Autodesk Fusion 360 part; units mm, degrees
note: some values were not read from the file. Set by a fixed rule: which face or edge a step refers to.
(part 4 of 12)
  spline S14 degree 5 poles (-2.4466, 3.8949) (-2.4467, 3.8949) (-2.4468, 3.8951) (-2.447, 3.8954) (-2.4473, 3.8958) (-2.4477, 3.8965) (-2.4482, 3.8972) (-2.4488, 3.8981) (-2.4495, 3.899) (-2.4502, 3.9) (-2.451, 3.9011) (-2.4518, 3.9023) (-2.4528, 3.9036) (-2.4538, 3.905) (-2.4549, 3.9065) (-2.456, 3.908) (-2.4572, 3.9096) (-2.4585, 3.9113) (-2.4599, 3.9131) (-2.4613, 3.9149) (-2.4629, 3.9168) (-2.4644, 3.9188) (-2.4661, 3.9208) (-2.4678, 3.9229) (-2.4696, 3.9251) (-2.4715, 3.9274) (-2.4734, 3.9297) (-2.4754, 3.9321) (-2.4775, 3.9345) (-2.4797, 3.937) (-2.4819, 3.9395) (-2.4842, 3.9421) (-2.4865, 3.9448) (-2.489, 3.9475) (-2.4915, 3.9503) (-2.4941, 3.9531) (-2.4967, 3.956) (-2.4994, 3.9589) (-2.5022, 3.9619) (-2.5051, 3.9649) (-2.508, 3.968) (-2.511, 3.9711) (-2.5141, 3.9742) (-2.5172, 3.9774) (-2.5205, 3.9807) (-2.5237, 3.9839) (-2.5271, 3.9873) (-2.5305, 3.9906) (-2.534, 3.994) (-2.5376, 3.9975) (-2.5412, 4.0009) (-2.5449, 4.0044) (-2.5487, 4.008) (-2.5525, 4.0116) (-2.5565, 4.0152) (-2.5604, 4.0188) (-2.5645, 4.0225) (-2.5686, 4.0262) (-2.5728, 4.0299) (-2.577, 4.0337) (-2.5814, 4.0375) (-2.5858, 4.0413) (-2.5902, 4.0451) (-2.5948, 4.049) (-2.5994, 4.0529) (-2.604, 4.0568) (-2.6088, 4.0607) (-2.6136, 4.0647) (-2.6184, 4.0686) (-2.6234, 4.0726) (-2.6284, 4.0767) (-2.6335, 4.0807) (-2.6386, 4.0848) (-2.6438, 4.0888) (-2.6491, 4.0929) (-2.6544, 4.097) (-2.6598, 4.1012) (-2.6653, 4.1053) (-2.6708, 4.1095) (-2.6764, 4.1136) (-2.6821, 4.1178) (-2.6878, 4.122) (-2.6936, 4.1262) (-2.6995, 4.1304) (-2.7055, 4.1346) (-2.7115, 4.1389) (-2.7175, 4.1431) (-2.7236, 4.1474) (-2.7298, 4.1516) (-2.7361, 4.1559) (-2.7424, 4.1602) (-2.7488, 4.1645) (-2.7553, 4.1688) (-2.7618, 4.1731) (-2.7684, 4.1774) (-2.775, 4.1817) (-2.7817, 4.186) (-2.7885, 4.1903) (-2.7953, 4.1946) (-2.8022, 4.1989) (-2.8092, 4.2032) (-2.8162, 4.2075) (-2.8233, 4.2119) (-2.8304, 4.2162) (-2.8376, 4.2205) (-2.8449, 4.2248) (-2.8522, 4.2291) (-2.8596, 4.2334) (-2.8671, 4.2377) (-2.8746, 4.2421) (-2.8822, 4.2464) (-2.8898, 4.2507) (-2.8975, 4.2549) (-2.9053, 4.2592) (-2.9131, 4.2635) (-2.921, 4.2678) (-2.9289, 4.2721) (-2.9369, 4.2763) (-2.945, 4.2806) (-2.9531, 4.2848) (-2.9613, 4.2891) (-2.9695, 4.2933) (-2.9778, 4.2975) (-2.9862, 4.3018) (-2.9946, 4.306) (-3.003, 4.3102) (-3.0116, 4.3143) (-3.0202, 4.3185) (-3.0288, 4.3227) (-3.0375, 4.3268) (-3.0463, 4.331) (-3.0551, 4.3351) (-3.064, 4.3392) (-3.0729, 4.3433) (-3.0819, 4.3474) (-3.0909, 4.3514) (-3.1, 4.3555) (-3.1092, 4.3595) (-3.1184, 4.3635) (-3.1277, 4.3676) (-3.137, 4.3715) (-3.1464, 4.3755) (-3.1558, 4.3795) (-3.1653, 4.3834) (-3.1749, 4.3873) (-3.1845, 4.3912) (-3.1941, 4.3951) (-3.2038, 4.399) (-3.2136, 4.4028) (-3.2234, 4.4067) (-3.2333, 4.4105) (-3.2432, 4.4143) (-3.2532, 4.418) (-3.2632, 4.4218) (-3.2733, 4.4255) (-3.2834, 4.4292) (-3.2936, 4.4329) (-3.3039, 4.4365) (-3.3141, 4.4402) (-3.3245, 4.4438) (-3.3349, 4.4474) (-3.3453, 4.4509) (-3.3558, 4.4545) (-3.3664, 4.458) (-3.377, 4.4615) (-3.3876, 4.465) (-3.3983, 4.4684) (-3.4091, 4.4718) (-3.4199, 4.4752) (-3.4307, 4.4786) (-3.4416, 4.4819) (-3.4526, 4.4853) (-3.4636, 4.4886) (-3.4746, 4.4918) (-3.4857, 4.495) (-3.4969, 4.4983) (-3.508, 4.5014) (-3.5193, 4.5046) (-3.5306, 4.5077) (-3.5419, 4.5108) (-3.5533, 4.5139) (-3.5647, 4.5169) (-3.5762, 4.5199) (-3.5877, 4.5229) (-3.5993, 4.5258) (-3.6109, 4.5287) (-3.6226, 4.5316) (-3.6343, 4.5345) (-3.646, 4.5373) (-3.6578, 4.5401) (-3.6697, 4.5429) (-3.6816, 4.5456) (-3.6935, 4.5483) (-3.7055, 4.5509) (-3.7175, 4.5536) (-3.7296, 4.5562) (-3.7417, 4.5587) (-3.7538, 4.5613) (-3.766, 4.5638) (-3.7783, 4.5662) (-3.7906, 4.5687) (-3.8029, 4.5711) (-3.8153, 4.5734) (-3.8277, 4.5757) (-3.8401, 4.578) (-3.8526, 4.5803) (-3.8652, 4.5825) (-3.8778, 4.5847) (-3.8904, 4.5868) (-3.903, 4.589) (-3.9157, 4.591) (-3.9285, 4.5931) (-3.9413, 4.5951) (-3.9541, 4.597) (-3.967, 4.599) (-3.9799, 4.6009) (-3.9928, 4.6027) (-4.0058, 4.6045) (-4.0188, 4.6063) (-4.0319, 4.6081) (-4.045, 4.6098) (-4.0582, 4.6114) (-4.0713, 4.6131) (-4.0846, 4.6146) (-4.0978, 4.6162) (-4.1111, 4.6177) (-4.1244, 4.6192) (-4.1378, 4.6206) (-4.1512, 4.622) (-4.1647, 4.6233) (-4.1782, 4.6246) (-4.1917, 4.6259) (-4.2052, 4.6271) (-4.2188, 4.6283) (-4.2324, 4.6295) (-4.2461, 4.6306) (-4.2598, 4.6316) (-4.2735, 4.6327) (-4.2873, 4.6336) (-4.3011, 4.6346) (-4.3149, 4.6355) (-4.326, 4.6362) (-4.3344, 4.6367) (-4.3399, 4.637) (-4.3427, 4.6371) knots 0 0 0 0 0 0 0.00416667 0.00833333 0.0125 0.01666667 0.02083333 0.025 0.02916667 0.03333333 0.0375 0.04166667 0.04583333 0.05 0.05416667 0.05833333 0.0625 0.06666667 0.07083333 0.075 0.07916667 0.08333333 0.0875 0.09166667 0.09583333 0.1 0.10416667 0.10833333 0.1125 0.11666667 0.12083333 0.125 0.12916667 0.13333333 0.1375 0.14166667 0.14583333 0.15 0.15416667 0.15833333 0.1625 0.16666667 0.17083333 0.175 0.17916667 0.18333333 0.1875 0.19166667 0.19583333 0.2 0.20416667 0.20833333 0.2125 0.21666667 0.22083333 0.225 0.22916667 0.23333333 0.2375 0.24166667 0.24583333 0.25 0.25416667 0.25833333 0.2625 0.26666667 0.27083333 0.275 0.27916667 0.28333333 0.2875 0.29166667 0.29583333 0.3 0.30416667 0.30833333 0.3125 0.31666667 0.32083333 0.325 0.32916667 0.33333333 0.3375 0.34166667 0.34583333 0.35 0.35416667 0.35833333 0.3625 0.36666667 0.37083333 0.375 0.37916667 0.38333333 0.3875 0.39166667 0.39583333 0.4 0.40416667 0.40833333 0.4125 0.41666667 0.42083333 0.425 0.42916667 0.43333333 0.4375 0.44166667 0.44583333 0.45 0.45416667 0.45833333 0.4625 0.46666667 0.47083333 0.475 0.47916667 0.48333333 0.4875 0.49166667 0.49583333 0.5 0.50416667 0.50833333 0.5125 0.51666667 0.52083333 0.525 0.52916667 0.53333333 0.5375 0.54166667 0.54583333 0.55 0.55416667 0.55833333 0.5625 0.56666667 0.57083333 0.575 0.57916667 0.58333333 0.5875 0.59166667 0.59583333 0.6 0.60416667 0.60833333 0.6125 0.61666667 0.62083333 0.625 0.62916667 0.63333333 0.6375 0.64166667 0.64583333 0.65 0.65416667 0.65833333 0.6625 0.66666667 0.67083333 0.675 0.67916667 0.68333333 0.6875 0.69166667 0.69583333 0.7 0.70416667 0.70833333 0.7125 0.71666667 0.72083333 0.725 0.72916667 0.73333333 0.7375 0.74166667 0.74583333 0.75 0.75416667 0.75833333 0.7625 0.76666667 0.77083333 0.775 0.77916667 0.78333333 0.7875 0.79166667 0.79583333 0.8 0.80416667 0.80833333 0.8125 0.81666667 0.82083333 0.825 0.82916667 0.83333333 0.8375 0.84166667 0.84583333 0.85 0.85416667 0.85833333 0.8625 0.86666667 0.87083333 0.875 0.87916667 0.88333333 0.8875 0.89166667 0.89583333 0.9 0.90416667 0.90833333 0.9125 0.91666667 0.92083333 0.925 0.92916667 0.93333333 0.9375 0.94166667 0.94583333 0.95 0.95416667 0.95833333 0.9625 0.96666667 0.97083333 0.975 0.97916667 0.98333333 0.9875 0.99166667 0.99583333 1 1 1 1 1 1
  arc A15 (-4.3427, 4.6371) -> (-4.6371, 4.3427) centre (0, 0) ccw
  spline S15 degree 5 poles (-4.6371, 4.3427) (-4.637, 4.3399) (-4.6367, 4.3344) (-4.6362, 4.326) (-4.6355, 4.3149) (-4.6346, 4.3011) (-4.6336, 4.2873) (-4.6327, 4.2735) (-4.6316, 4.2598) (-4.6306, 4.2461) (-4.6295, 4.2324) (-4.6283, 4.2188) (-4.6271, 4.2052) (-4.6259, 4.1917) (-4.6246, 4.1782) (-4.6233, 4.1647) (-4.622, 4.1512) (-4.6206, 4.1378) (-4.6192, 4.1244) (-4.6177, 4.1111) (-4.6162, 4.0978) (-4.6146, 4.0846) (-4.6131, 4.0713) (-4.6114, 4.0582) (-4.6098, 4.045) (-4.6081, 4.0319) (-4.6063, 4.0188) (-4.6045, 4.0058) (-4.6027, 3.9928) (-4.6009, 3.9799) (-4.599, 3.967) (-4.597, 3.9541) (-4.5951, 3.9413) (-4.5931, 3.9285) (-4.591, 3.9157) (-4.589, 3.903) (-4.5868, 3.8904) (-4.5847, 3.8778) (-4.5825, 3.8652) (-4.5803, 3.8526) (-4.578, 3.8401) (-4.5757, 3.8277) (-4.5734, 3.8153) (-4.5711, 3.8029) (-4.5687, 3.7906) (-4.5662, 3.7783) (-4.5638, 3.766) (-4.5613, 3.7538) (-4.5587, 3.7417) (-4.5562, 3.7296) (-4.5536, 3.7175) (-4.5509, 3.7055) (-4.5483, 3.6935) (-4.5456, 3.6816) (-4.5429, 3.6697) (-4.5401, 3.6578) (-4.5373, 3.646) (-4.5345, 3.6343) (-4.5316, 3.6226) (-4.5287, 3.6109) (-4.5258, 3.5993) (-4.5229, 3.5877) (-4.5199, 3.5762) (-4.5169, 3.5647) (-4.5139, 3.5533) (-4.5108, 3.5419) (-4.5077, 3.5306) (-4.5046, 3.5193) (-4.5014, 3.508) (-4.4983, 3.4969) (-4.495, 3.4857) (-4.4918, 3.4746) (-4.4886, 3.4636) (-4.4853, 3.4526) (-4.4819, 3.4416) (-4.4786, 3.4307) (-4.4752, 3.4199) (-4.4718, 3.4091) (-4.4684, 3.3983) (-4.465, 3.3876) (-4.4615, 3.377) (-4.458, 3.3664) (-4.4545, 3.3558) (-4.4509, 3.3453) (-4.4474, 3.3349) (-4.4438, 3.3245) (-4.4402, 3.3141) (-4.4365, 3.3039) (-4.4329, 3.2936) (-4.4292, 3.2834) (-4.4255, 3.2733) (-4.4218, 3.2632) (-4.418, 3.2532) (-4.4143, 3.2432) (-4.4105, 3.2333) (-4.4067, 3.2234) (-4.4028, 3.2136) (-4.399, 3.2038) (-4.3951, 3.1941) (-4.3912, 3.1845) (-4.3873, 3.1749) (-4.3834, 3.1653) (-4.3795, 3.1558) (-4.3755, 3.1464) (-4.3715, 3.137) (-4.3676, 3.1277) (-4.3635, 3.1184) (-4.3595, 3.1092) (-4.3555, 3.1) (-4.3514, 3.0909) (-4.3474, 3.0819) (-4.3433, 3.0729) (-4.3392, 3.064) (-4.3351, 3.0551) (-4.331, 3.0463) (-4.3268, 3.0375) (-4.3227, 3.0288) (-4.3185, 3.0202) (-4.3143, 3.0116) (-4.3102, 3.003) (-4.306, 2.9946) (-4.3018, 2.9862) (-4.2975, 2.9778) (-4.2933, 2.9695) (-4.2891, 2.9613) (-4.2848, 2.9531) (-4.2806, 2.945) (-4.2763, 2.9369) (-4.2721, 2.9289) (-4.2678, 2.921) (-4.2635, 2.9131) (-4.2592, 2.9053) (-4.2549, 2.8975) (-4.2507, 2.8898) (-4.2464, 2.8822) (-4.2421, 2.8746) (-4.2377, 2.8671) (-4.2334, 2.8596) (-4.2291, 2.8522) (-4.2248, 2.8449) (-4.2205, 2.8376) (-4.2162, 2.8304) (-4.2119, 2.8233) (-4.2075, 2.8162) (-4.2032, 2.8092) (-4.1989, 2.8022) (-4.1946, 2.7953) (-4.1903, 2.7885) (-4.186, 2.7817) (-4.1817, 2.775) (-4.1774, 2.7684) (-4.1731, 2.7618) (-4.1688, 2.7553) (-4.1645, 2.7488) (-4.1602, 2.7424) (-4.1559, 2.7361) (-4.1516, 2.7298) (-4.1474, 2.7236) (-4.1431, 2.7175) (-4.1389, 2.7115) (-4.1346, 2.7055) (-4.1304, 2.6995) (-4.1262, 2.6936) (-4.122, 2.6878) (-4.1178, 2.6821) (-4.1136, 2.6764) (-4.1095, 2.6708) (-4.1053, 2.6653) (-4.1012, 2.6598) (-4.097, 2.6544) (-4.0929, 2.6491) (-4.0888, 2.6438) (-4.0848, 2.6386) (-4.0807, 2.6335) (-4.0767, 2.6284) (-4.0726, 2.6234) (-4.0686, 2.6184) (-4.0647, 2.6136) (-4.0607, 2.6088) (-4.0568, 2.604) (-4.0529, 2.5994) (-4.049, 2.5948) (-4.0451, 2.5902) (-4.0413, 2.5858) (-4.0375, 2.5814) (-4.0337, 2.577) (-4.0299, 2.5728) (-4.0262, 2.5686) (-4.0225, 2.5645) (-4.0188, 2.5604) (-4.0152, 2.5565) (-4.0116, 2.5525) (-4.008, 2.5487) (-4.0044, 2.5449) (-4.0009, 2.5412) (-3.9975, 2.5376) (-3.994, 2.534) (-3.9906, 2.5305) (-3.9873, 2.5271) (-3.9839, 2.5237) (-3.9807, 2.5205) (-3.9774, 2.5172) (-3.9742, 2.5141) (-3.9711, 2.511) (-3.968, 2.508) (-3.9649, 2.5051) (-3.9619, 2.5022) (-3.9589, 2.4994) (-3.956, 2.4967) (-3.9531, 2.4941) (-3.9503, 2.4915) (-3.9475, 2.489) (-3.9448, 2.4865) (-3.9421, 2.4842) (-3.9395, 2.4819) (-3.937, 2.4797) (-3.9345, 2.4775) (-3.9321, 2.4754) (-3.9297, 2.4734) (-3.9274, 2.4715) (-3.9251, 2.4696) (-3.9229, 2.4678) (-3.9208, 2.4661) (-3.9188, 2.4644) (-3.9168, 2.4629) (-3.9149, 2.4613) (-3.9131, 2.4599) (-3.9113, 2.4585) (-3.9096, 2.4572) (-3.908, 2.456) (-3.9065, 2.4549) (-3.905, 2.4538) (-3.9036, 2.4528) (-3.9023, 2.4518) (-3.9011, 2.451) (-3.9, 2.4502) (-3.899, 2.4495) (-3.8981, 2.4488) (-3.8972, 2.4482) (-3.8965, 2.4477) (-3.8958, 2.4473) (-3.8954, 2.447) (-3.8951, 2.4468) (-3.8949, 2.4467) (-3.8949, 2.4466) knots -1 -1 -1 -1 -1 -1 -0.99583333 -0.99166667 -0.9875 -0.98333333 -0.97916667 -0.975 -0.97083333 -0.96666667 -0.9625 -0.95833333 -0.95416667 -0.95 -0.94583333 -0.94166667 -0.9375 -0.93333333 -0.92916667 -0.925 -0.92083333 -0.91666667 -0.9125 -0.90833333 -0.90416667 -0.9 -0.89583333 -0.89166667 -0.8875 -0.88333333 -0.87916667 -0.875 -0.87083333 -0.86666667 -0.8625 -0.85833333 -0.85416667 -0.85 -0.84583333 -0.84166667 -0.8375 -0.83333333 -0.82916667 -0.825 -0.82083333 -0.81666667 -0.8125 -0.80833333 -0.80416667 -0.8 -0.79583333 -0.79166667 -0.7875 -0.78333333 -0.77916667 -0.775 -0.77083333 -0.76666667 -0.7625 -0.75833333 -0.75416667 -0.75 -0.74583333 -0.74166667 -0.7375 -0.73333333 -0.72916667 -0.725 -0.72083333 -0.71666667 -0.7125 -0.70833333 -0.70416667 -0.7 -0.69583333 -0.69166667 -0.6875 -0.68333333 -0.67916667 -0.675 -0.67083333 -0.66666667 -0.6625 -0.65833333 -0.65416667 -0.65 -0.64583333 -0.64166667 -0.6375 -0.63333333 -0.62916667 -0.625 -0.62083333 -0.61666667 -0.6125 -0.60833333 -0.60416667 -0.6 -0.59583333 -0.59166667 -0.5875 -0.58333333 -0.57916667 -0.575 -0.57083333 -0.56666667 -0.5625 -0.55833333 -0.55416667 -0.55 -0.54583333 -0.54166667 -0.5375 -0.53333333 -0.52916667 -0.525 -0.52083333 -0.51666667 -0.5125 -0.50833333 -0.50416667 -0.5 -0.49583333 -0.49166667 -0.4875 -0.48333333 -0.47916667 -0.475 -0.47083333 -0.46666667 -0.4625 -0.45833333 -0.45416667 -0.45 -0.44583333 -0.44166667 -0.4375 -0.43333333 -0.42916667 -0.425 -0.42083333 -0.41666667 -0.4125 -0.40833333 -0.40416667 -0.4 -0.39583333 -0.39166667 -0.3875 -0.38333333 -0.37916667 -0.375 -0.37083333 -0.36666667 -0.3625 -0.35833333 -0.35416667 -0.35 -0.34583333 -0.34166667 -0.3375 -0.33333333 -0.32916667 -0.325 -0.32083333 -0.31666667 -0.3125 -0.30833333 -0.30416667 -0.3 -0.29583333 -0.29166667 -0.2875 -0.28333333 -0.27916667 -0.275 -0.27083333 -0.26666667 -0.2625 -0.25833333 -0.25416667 -0.25 -0.24583333 -0.24166667 -0.2375 -0.23333333 -0.22916667 -0.225 -0.22083333 -0.21666667 -0.2125 -0.20833333 -0.20416667 -0.2 -0.19583333 -0.19166667 -0.1875 -0.18333333 -0.17916667 -0.175 -0.17083333 -0.16666667 -0.1625 -0.15833333 -0.15416667 -0.15 -0.14583333 -0.14166667 -0.1375 -0.13333333 -0.12916667 -0.125 -0.12083333 -0.11666667 -0.1125 -0.10833333 -0.10416667 -0.1 -0.09583333 -0.09166667 -0.0875 -0.08333333 -0.07916667 -0.075 -0.07083333 -0.06666667 -0.0625 -0.05833333 -0.05416667 -0.05 -0.04583333 -0.04166667 -0.0375 -0.03333333 -0.02916667 -0.025 -0.02083333 -0.01666667 -0.0125 -0.00833333 -0.00416667 0 0 0 0 0 0
  line L30 (-3.8949, 2.4466) -> (-3.8941, 2.4462)
  line L31 (-3.8941, 2.4462) -> (-3.1172, 1.9582)
  circle A16 centre (0, 0) radius 2.925
  line L32 (3, 1) -> (-3, 1)
  line L33 (-3, 1) -> (-3, -1)
  line L34 (-3, -1) -> (3, -1)
  line L35 (3, -1) -> (3, 1)
  line L36 (3, 1) -> (-3, -1) construction
  line L37 (-3, 1) -> (3, -1) construction
  line L38 (2.9, 0.9) -> (-2.9, 0.9)
  line L39 (-2.9, 0.9) -> (-2.9, -0.9)
  line L40 (-2.9, -0.9) -> (2.9, -0.9)
  line L41 (2.9, -0.9) -> (2.9, 0.9)
  line L42 (0, -1) -> (0, 1)
  dimension "d32" = 5.85
  dimension "d37" = 6
  dimension "d38" = 2
  dimension "d39" = -0.1
  constraint concentric A0 A16
  constraint horizontal L32
  constraint perpendicular L32 L33
  constraint parallel L32 L34
  constraint parallel L33 L35
  constraint coincident L36 A0.centre
  constraint coincident L37 A0.centre
  constraint coincident A0.centre A1.centre
  constraint midpoint L34 L42.start
  constraint midpoint L32 L42.end
  measures "d32" diameter of A16
  measures "d37" distance of L33.end L34.end
  measures "d38" distance of L32.end L33.end
extrude "Extrude4" cut sketch "Sketch2 (3)" against normal blind 5 contours A16 L32 L38 L42 | A16 L34 L40 L42 | A16 L32 | A16 L38 L39 L40 L42 | A16 L32 L38 L42 | A16 L34 | A16 L34 L40 L42 | A16 L39 bodies 1 in component "Component"
extrude "Extrude3" cut sketch "Sketch2 (3)" against normal blind 5 contours A16 L32 L38 L42 | A16 L34 L40 L42 | A16 L32 | A16 L38 L39 L40 L42 | A16 L32 L38 L42 | A16 L34 | A16 L34 L40 L42 | A16 L39 bodies 10 in component "Component'"
component "Component" placed x (1, 0, 0) y (0, 1, 0) z (0, 0, 1) at (30, 0, 0)
component "Component'" placed x (1, 0, 0) y (0, 1, 0) z (0, 0, 1) at (0, 0, 0)
component "Component" placed x (1, 0, 0) y (0, 1, 0) z (0, 0, 1) at (45, 0, 0)
component "Component'" placed x (1, 0, 0) y (0, 1, 0) z (0, 0, 1) at (-46, 0, 0)

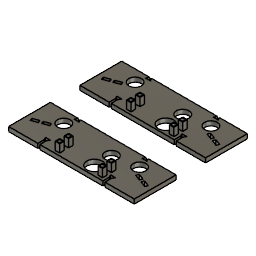
design "card-shuffler-side-plates"
part number: 2026-07-14-13-37-18-342
part number: 2026-07-29-15-30-40-937
Autodesk Fusion 360 part; units mm, degrees
sketch "Sketch1" plane through (0, 0, 0) normal (0, 0, 1) x (1, 0, 0)
  line L0 (0, 0) -> (81, 0)
  line L1 (81, 0) -> (81, 103)
  line L2 (81, 103) -> (0, 103)
  line L3 (0, 103) -> (0, 0)
  line L4 (76, 98) -> (5, 98)
  line L5 (5, 98) -> (5, 5)
  line L6 (5, 5) -> (76, 5)
  line L7 (76, 5) -> (76, 98)
  line L8 (76, 98) -> (5, 5) construction
  line L9 (5, 98) -> (76, 5) construction
  line L10 (81, 0) -> (111, 0)
  line L11 (111, 0) -> (111, 5)
  line L12 (111, 5) -> (81, 5)
  line L13 (81, 5) -> (81, 0)
  line L14 (0, 0) -> (-30, 0)
  line L15 (-30, 0) -> (-30, 5)
  line L16 (-30, 5) -> (0, 5)
  line L17 (0, 5) -> (0, 0)
  line L18 (81, 103) -> (111, 103)
  line L19 (111, 103) -> (111, 98)
  line L20 (111, 98) -> (81, 98)
  line L21 (81, 98) -> (81, 103)
  line L22 (0, 103) -> (-30, 103)
  line L23 (-30, 103) -> (-30, 98)
  line L24 (-30, 98) -> (0, 98)
  line L25 (0, 98) -> (0, 103)
  line L26 (76, 51.5) -> (76, 45)
  line L27 (76, 45) -> (81, 45)
  line L28 (81, 45) -> (81, 58)
  line L29 (81, 58) -> (76, 58)
  line L30 (76, 58) -> (76, 45)
  line L31 (0, 58) -> (5, 58)
  line L32 (5, 58) -> (5, 45)
  line L33 (5, 45) -> (0, 45)
  line L34 (0, 45) -> (0, 58)
  line L35 (81, 98) -> (111, 98)
  line L36 (111, 98) -> (111, 5)
  line L37 (111, 5) -> (81, 5)
  line L38 (81, 5) -> (81, 98)
  line L39 (-30, 98) -> (0, 98)
  line L40 (0, 98) -> (0, 5)
  line L41 (0, 5) -> (-30, 5)
  line L42 (-30, 5) -> (-30, 98)
  line L43 (76, 58) -> (108, 58)
  line L44 (108, 58) -> (108, 45)
  line L45 (108, 45) -> (76, 45)
  line L46 (76, 45) -> (76, 58)
  line L47 (5, 45) -> (-27, 45)
  line L48 (-27, 45) -> (-27, 58)
  line L49 (-27, 58) -> (5, 58)
  line L50 (5, 58) -> (5, 45)
  line L51 (76, 98) -> (81, 98)
  line L52 (5, 98) -> (0, 98)
  line L53 (0, 5) -> (5, 5)
  line L54 (76, 5) -> (81, 5)
  point P0 (40.5, 51.5)
  dimension "d1" = 81
  dimension "d2" = 103
  dimension "d3" = 71
  dimension "d4" = 93
  dimension "d7" = 6.5
  dimension "d8" = 32
  dimension "d9" = 13
  dimension "d14" = 30
  dimension "d15" = 30
  dimension "d16" = 30
  dimension "d17" = 30
  constraint horizontal L0
  constraint vertical L1
  constraint horizontal L2
  constraint vertical L3
  constraint coincident L0.start L3.end
  constraint horizontal L4
  constraint perpendicular L4 L5
  constraint parallel L4 L6
  constraint parallel L5 L7
  constraint coincident L8 P0
  constraint coincident L9 P0
  constraint horizontal L10
  constraint vertical L11
  constraint horizontal L12
  constraint vertical L13
  constraint horizontal L14
  constraint vertical L15
  constraint horizontal L16
  constraint vertical L17
  constraint horizontal L18
  constraint vertical L19
  constraint horizontal L20
  constraint vertical L21
  constraint horizontal L22
  constraint vertical L23
  constraint horizontal L24
  constraint vertical L25
  constraint midpoint L7 L26.start
  constraint parallel L7 L26
  constraint horizontal L27
  constraint vertical L28
  constraint horizontal L29
  constraint vertical L30
  constraint coincident L1 L28.end
  constraint horizontal L31
  constraint vertical L32
  constraint horizontal L33
  constraint vertical L34
  constraint coincident L5 L32.end
  constraint coincident L3 L31.start
  constraint horizontal L35
  constraint vertical L36
  constraint horizontal L37
  constraint vertical L38
  constraint horizontal L39
  constraint vertical L40
  constraint horizontal L41
  constraint vertical L42
  constraint horizontal L43
  constraint vertical L44
  constraint horizontal L45
  constraint vertical L46
  constraint horizontal L47
  constraint vertical L48
  constraint horizontal L49
  constraint vertical L50
  measures "d1" distance of L0.start L0.end
  measures "d2" distance of L0.start L2.end
  measures "d3" distance of L5.end L6.end
  measures "d4" distance of L4.end L5.end
  measures "d7" distance of L26.start L26.end
  measures "d8" distance of L32.end L47.end
  measures "d9" distance of L32.end L31.end
  measures "d14" distance of L36 L38
  measures "d15" distance of L3 L42
  measures "d16" distance of L15 L17
  measures "d17" distance of L19 L21
extrude "Extrude1" add sketch "Sketch1" along normal blind 62 contours L0 L1 L3 L6 L13 L17 L53 L54 | L3 L14 L15 L16 L17 L41 | L1 L10 L11 L12 L13 L37 makes body 1
sketch "Sketch2" plane through (0, 0, 62) normal (0, 0, 1) x (-1, 0, 0)
  line L0 (-76, -98) -> (-81, -98)
  line L1 (-5, -98) -> (0, -98)
  line L2 (0, -5) -> (-5, -5)
  line L3 (40, -98) -> (-121, -98)
  line L4 (-121, -98) -> (-121, -103)
  line L5 (-121, -103) -> (40, -103)
  line L6 (40, -103) -> (40, -98)
  line L7 (40, -5) -> (-121, -5)
  line L8 (-121, -5) -> (-121, 0)
  line L9 (-121, 0) -> (40, 0)
  line L10 (40, 0) -> (40, -5)
  line L11 (0, -5) -> (30, -5)
  line L12 (30, -5) -> (30, 0)
  line L13 (30, 0) -> (-111, 0)
  line L14 (-111, 0) -> (-111, -5)
  line L15 (-111, -5) -> (-81, -5)
  line L16 (-81, -5) -> (-76, -5)
  line L17 (-76, -5) -> (-5, -5)
  line L18 (-5, -5) -> (0, -5)
  constraint horizontal L3
  constraint vertical L4
  constraint horizontal L5
  constraint vertical L6
  constraint horizontal L7
  constraint vertical L8
  constraint horizontal L9
  constraint vertical L10
sketch "Sketch5" plane through (0, 0, 0) normal (0, -1, 0) x (1, 0, 0)
  line L0 (-30, 0) -> (111, 0)
  line L1 (111, 0) -> (111, 62)
  line L2 (111, 62) -> (-30, 62)
  line L3 (-30, 62) -> (-30, 0)
  line L4 (40.5, 62) -> (40.5, 0)
  circle A0 centre (-2, 28) radius 7.05
  circle A1 centre (56, 51.6) radius 8.5
  circle A2 centre (70, 46.6) radius 1.95
  circle A3 centre (70, 56.6) radius 1.95
  line L5 (72.5, 59.1) -> (67.5, 59.1)
  line L6 (67.5, 59.1) -> (67.5, 54.1)
  line L7 (67.5, 54.1) -> (72.5, 54.1)
  line L8 (72.5, 54.1) -> (72.5, 59.1)
  line L9 (72.5, 59.1) -> (67.5, 54.1) construction
  line L10 (67.5, 59.1) -> (72.5, 54.1) construction
  line L11 (72.5, 49.1) -> (67.5, 49.1)
  line L12 (67.5, 49.1) -> (67.5, 44.1)
  line L13 (67.5, 44.1) -> (72.5, 44.1)
  line L14 (72.5, 44.1) -> (72.5, 49.1)
  line L15 (72.5, 49.1) -> (67.5, 44.1) construction
  line L16 (67.5, 49.1) -> (72.5, 44.1) construction
  circle A4 centre (83, 28) radius 7.05
  line L17 (0, 0) -> (80, 0)
  line L18 (80, 0) -> (80, 15)
  line L19 (80, 15) -> (0, 15)
  line L20 (0, 15) -> (0, 0)
  line L21 (0, 15) -> (-30, 15)
  line L22 (-30, 15) -> (-30, 0)
  line L23 (-30, 0) -> (0, 0)
  line L24 (0, 0) -> (0, 15)
  line L25 (80, 15) -> (111, 15)
  line L26 (111, 15) -> (111, 0)
  line L27 (111, 0) -> (80, 0)
  line L28 (80, 0) -> (80, 15)
  line L29 (0, 15) -> (5, 15)
  line L30 (5, 15) -> (5, 18)
  line L31 (5, 18) -> (0, 18)
  line L32 (0, 18) -> (0, 15)
  line L33 (80, 15) -> (75, 15)
  line L34 (81, 18) -> (76, 18)
  line L35 (76, 18) -> (76, 15)
  line L36 (76, 15) -> (81, 15)
  line L37 (81, 15) -> (81, 18)
  line L38 (-7.7431, 38.0574) -> (-14.3209, 40.4516)
  line L39 (-7.7431, 38.0574) -> (-8.7691, 35.2384)
  line L40 (-8.7691, 35.2384) -> (-15.347, 37.6325)
  line L41 (-15.347, 37.6325) -> (-14.3209, 40.4516)
  line L42 (-17.1354, 41.4902) -> (-23.7133, 43.8843)
  line L43 (-17.1354, 41.4902) -> (-18.1615, 38.6711)
  line L44 (-18.1615, 38.6711) -> (-24.7393, 41.0652)
  line L45 (-24.7393, 41.0652) -> (-23.7133, 43.8843)
  line L46 (105.7393, 41.0652) -> (104.7133, 43.8843)
  line L47 (99.1615, 38.6711) -> (105.7393, 41.0652)
  line L48 (96.347, 37.6325) -> (95.3209, 40.4516)
  line L49 (88.7431, 38.0574) -> (95.3209, 40.4516)
  line L50 (98.1354, 41.4902) -> (99.1615, 38.6711)
  line L51 (98.1354, 41.4902) -> (104.7133, 43.8843)
  line L52 (89.7691, 35.2384) -> (96.347, 37.6325)
  line L53 (88.7431, 38.0574) -> (89.7691, 35.2384)
  line L54 (19.5, 59.1) -> (19.5, 54.1)
  line L55 (24.5, 49.1) -> (19.5, 49.1)
  line L56 (24.5, 44.1) -> (24.5, 49.1)
  line L57 (19.5, 44.1) -> (24.5, 44.1)
  line L58 (19.5, 49.1) -> (24.5, 44.1) construction
  line L59 (24.5, 59.1) -> (19.5, 59.1)
  line L60 (24.5, 54.1) -> (24.5, 59.1)
  line L61 (19.5, 54.1) -> (24.5, 54.1)
  line L62 (24.5, 59.1) -> (19.5, 54.1) construction
  circle A5 centre (22, 56.6) radius 1.95
  line L63 (19.5, 49.1) -> (19.5, 44.1)
  line L64 (19.5, 59.1) -> (24.5, 54.1) construction
  circle A6 centre (22, 46.6) radius 1.95
  line L65 (24.5, 49.1) -> (19.5, 44.1) construction
  line L66 (75, 62) -> (75, 36)
  line L67 (104.7133, 43.8843) -> (40.5, 20.5126)
  line L68 (40.5, 20.5126) -> (-23.7133, 43.8843)
  line L69 (62, 62) -> (62, 42)
  circle A7 centre (56, 32.6) radius 7.05
  line L70 (0, 18) -> (2.5, 13.6699)
  line L71 (2.5, 13.6699) -> (5, 18)
  line L72 (5, 18) -> (0, 18)
  line L73 (76, 18) -> (78.5, 13.6699)
  line L74 (78.5, 13.6699) -> (81, 18)
  line L75 (81, 18) -> (76, 18)
  line L76 (5.2598, 18.15) -> (-0.2598, 18.15)
  line L77 (-0.2598, 18.15) -> (2.5, 13.3699)
  line L78 (2.5, 13.3699) -> (5.2598, 18.15)
  line L79 (75.7402, 18.15) -> (78.5, 13.3699)
  line L80 (78.5, 13.3699) -> (81.2598, 18.15)
  line L81 (81.2598, 18.15) -> (75.7402, 18.15)
  point P0 (106, 74)
  point P1 (70, 56.6)
  point P2 (70, 46.6)
  point P3 (22, 46.6)
  point P4 (22, 56.6)
  point P5 (2.5, 16.5566)
  point P6 (78.5, 16.5566)
  dimension "d91" = 14.1
  dimension "d93" = 28
  dimension "d97" = 28
  dimension "d98" = 17
  dimension "d100" = 10.4
  dimension "d101" = 3.9
  dimension "d102" = 3.9
  dimension "d104" = 5
  dimension "d106" = 5
  dimension "d107" = 5
  dimension "d108" = 5
  dimension "d109" = 5
  dimension "d110" = 5
  dimension "d117" = 7
  dimension "d120" = 3
  dimension "d121" = 7
  dimension "d122" = 7
  dimension "d124" = 3
  dimension "d125" = 7
  dimension "d126" = 3
  dimension "d127" = 3.9
  dimension "d128" = 3.9
  dimension "d129" = 5
  dimension "d130" = 5
  dimension "d131" = 5
  dimension "d132" = 5
  dimension "d135" = 3
  dimension "d136" = 3
  dimension "d145" = 14
  dimension "d146" = 14
  dimension "d147" = 14.1
  dimension "d149" = 19
  dimension "d154" = 0.15
  constraint midpoint L2 L4.start
  constraint midpoint L0 L4.end
  constraint horizontal L5
  constraint perpendicular L5 L6
  constraint parallel L5 L7
  constraint parallel L6 L8
  constraint coincident L9 P1
  constraint coincident L10 P1
  constraint coincident P1 A3.centre
  constraint horizontal L11
  constraint perpendicular L11 L12
  constraint parallel L11 L13
  constraint parallel L12 L14
  constraint coincident L15 P2
  constraint coincident L16 P2
  constraint coincident P2 A2.centre
  constraint symmetric L4 A0 A4
  constraint horizontal L17
  constraint vertical L18
  constraint horizontal L19
  constraint vertical L20
  constraint coincident L17.start L20.end
  constraint horizontal L21
  constraint vertical L22
  constraint horizontal L23
  constraint vertical L24
  constraint coincident L0.start L3.end
  constraint horizontal L25
  constraint vertical L26
  constraint horizontal L27
  constraint vertical L28
  constraint coincident L0.end L1.start
  constraint horizontal L29
  constraint vertical L30
  constraint horizontal L31
  constraint vertical L32
  constraint horizontal L33
  constraint horizontal L34
  constraint vertical L35
  constraint horizontal L36
  constraint vertical L37
  constraint coincident L19 L35.end
  constraint perpendicular L38 L39
  constraint perpendicular L39 L40
  constraint perpendicular L41 L42
  constraint perpendicular L42 L43
  constraint perpendicular L43 L44
  constraint symmetric L4 L38.start L49.start
  constraint symmetric L4 L38.end L48.end
  constraint symmetric L4 L39.end L52.start
  constraint symmetric L4 L40.end L48.start
  constraint symmetric L4 L42.start L50.start
  constraint symmetric L4 L42.end L46.end
  constraint symmetric L4 L43.end L47.start
  constraint symmetric L4 L44.end L46.start
  constraint horizontal L59
  constraint perpendicular L54 L59
  constraint parallel L59 L61
  constraint parallel L54 L60
  constraint coincident P4 L62
  constraint coincident P4 L64
  constraint coincident P4 A5.centre
  constraint horizontal L55
  constraint perpendicular L55 L63
  constraint parallel L55 L57
  constraint parallel L56 L63
  constraint coincident P3 L65
  constraint coincident P3 L58
  constraint coincident P3 A6.centre
  constraint coincident L2 L66.start
  constraint perpendicular L2 L66
  constraint coincident L4 L67.end
  constraint perpendicular L48 L67
  constraint coincident L2 L69.start
  constraint perpendicular L2 L69
  measures "d91" diameter of A0
  measures "d93" distance of L0 A0.centre
  measures "d97" distance of L3 A0.centre
  measures "d98" diameter of A1
  measures "d100" distance of L2 A1.centre
  measures "d101" diameter of A2
  measures "d102" diameter of A3
  measures "d104" distance of A1.centre P1
  measures "d106" distance of A1.centre P2
  measures "d107" distance of L6.end L7.end
  measures "d108" distance of L5.end L6.end
  measures "d109" distance of L12.end L13.end
  measures "d110" distance of L11.end L12.end
  measures "d117" distance of L38.start L38.end
  measures "d120" distance of L38.start L39.end
  measures "d121" distance of L39.end L40.end
  measures "d122" distance of L42.start L42.end
  measures "d124" distance of L42.start L43.end
  measures "d125" distance of L43.end L44.end
  measures "d126" distance of L41 L43
  measures "d127" diameter of A6
  measures "d128" diameter of A5
  measures "d129" distance of L54.end L60.start
  measures "d130" distance of L54.end L54.start
  measures "d131" distance of L57.start L56.start
  measures "d132" distance of L55.end L57.start
  measures "d135" distance of L19.end L31.end
  measures "d136" distance of L34.end L35.end
  measures "d145" distance of A1.centre P1
  measures "d146" distance of A1.centre P2
  measures "d147" diameter of A7
  measures "d149" distance of A1.centre A7.centre
ref_plane "WorkPlane2" through (40.5, 2.5, 31) normal (1, 0, 0) x (0, 1, 0)
extrude "Extrude13" cut sketch "Sketch5" against normal blind 5 contours L0 L3 L20 L21 L22 L23 L24 | L0 L4 L17 L19 L20 L24 L29 L77 L78 | L0 L4 L17 L18 L19 L28 L33 L36 L79 L80 | L0 L1 L18 L25 L26 L27 L28 L36 | L19 L29 L32 L70 L77 | L19 L29 L70 L71 L77 L78 | L30 L31 L32 L72 L76 L77 L78 | L19 L29 L31 L70 L71 L72 | L19 L29 L70 L71 | L19 L33 L36 L73 L74 L79 L80 | L19 L33 L36 L37 L74 L80 | L19 L29 L30 L71 L78 | L19 L33 L36 L73 L74 | L19 L33 L34 L36 L73 L74 L75 | L34 L35 L37 L75 L79 L80 L81 | L19 L33 L35 L36 L73 L79 | A0 | A1 L69 | A1 L69 | A2 | A3 | L5 L6 L7 L8 | L11 L12 L13 L14 | A4 | L38 L39 L40 L41 | L42 L43 L44 L45 L68 | L46 L47 L50 L51 L67 | L48 L49 L52 L53 | A5 | A6 | L67 A7 | L67 A7 bodies 1
delete_face "DeleteFace1" 4 faces at (76.5196, 5, 15.9) (79.0137, 5, 19.3003) (79.3333, 5, 52.9201) (80.4804, 5, 15.9) on bodies 1
delete_face "DeleteFace2" 1 faces at (1.6667, 5, 52.9201) on bodies 1
copy_body "Body->Comp2" bodies 1 removing the originals makes body 2 in component "Component"
extrude "Extrude2" add sketch "Sketch5" against normal blind 14 contours L5 L6 L7 L8 | L11 L12 L13 L14 | L54 L59 L60 L61 | L55 L56 L57 L63 bodies 2 in component "Component"
sketch "Sketch8" plane through (0, 0, 62) normal (0, 0, 1) x (-1, 0, 0)
  line L0 (-111, -5) -> (30, -5)
  line L1 (30, -5) -> (30, 0)
  line L2 (30, 0) -> (-111, 0)
  line L3 (-81, 0) -> (-76, 0)
  line L4 (-76, 0) -> (-76, -5)
  line L5 (-76, -5) -> (-81, -5)
  line L6 (-81, -5) -> (-81, 0)
  line L7 (0, 0) -> (-5, 0)
  line L8 (-5, 0) -> (-5, -5)
  line L9 (-5, -5) -> (0, -5)
  line L10 (0, -5) -> (0, 0)
  line L11 (-111, 0) -> (-111, -5)
  line L12 (-5, 0) -> (-3, 0)
  line L13 (-3, 0) -> (-3, -5)
  line L14 (-3, -5) -> (-5, -5)
  line L15 (-5, -5) -> (-5, 0)
  line L16 (-76, -5) -> (-78, -5)
  line L17 (-78, -5) -> (-78, 0)
  line L18 (-78, 0) -> (-76, 0)
  line L19 (-76, 0) -> (-76, -5)
  line L20 (-5.5, -5) -> (-2.5, -5)
  line L21 (-2.5, -5) -> (-2.5, 0)
  line L22 (-2.5, 0) -> (-5.5, 0)
  line L23 (-5.5, 0) -> (-5.5, -5)
  line L24 (-5.5, -5) -> (-2.5, 0) construction
  line L25 (-2.5, -5) -> (-5.5, 0) construction
  line L26 (-78.5, -5) -> (-75.5, -5)
  line L27 (-75.5, -5) -> (-75.5, 0)
  line L28 (-75.5, 0) -> (-78.5, 0)
  line L29 (-78.5, 0) -> (-78.5, -5)
  line L30 (-78.5, -5) -> (-75.5, 0) construction
  line L31 (-75.5, -5) -> (-78.5, 0) construction
  line L32 (-75.9, 0) -> (-78.1, 0)
  line L33 (-78.1, 0) -> (-78.1, -5)
  line L34 (-78.1, -5) -> (-75.9, -5)
  line L35 (-75.9, -5) -> (-75.9, 0)
  line L36 (-75.9, 0) -> (-78.1, -5) construction
  line L37 (-78.1, 0) -> (-75.9, -5) construction
  line L38 (-2.9, 0) -> (-5.1, 0)
  line L39 (-5.1, 0) -> (-5.1, -5)
  line L40 (-5.1, -5) -> (-2.9, -5)
  line L41 (-2.9, -5) -> (-2.9, 0)
  line L42 (-2.9, 0) -> (-5.1, -5) construction
  line L43 (-5.1, 0) -> (-2.9, -5) construction
  point P0 (-2.5, -2.5)
  point P1 (-78.5, -2.5)
  point P2 (-4, -2.5)
  point P3 (-77, -2.5)
  point P4 (-77, -2.5)
  point P5 (-4, -2.5)
  constraint horizontal L3
  constraint vertical L4
  constraint horizontal L5
  constraint vertical L6
  constraint coincident L0 L4.end
  constraint coincident L2 L3.start
  constraint horizontal L7
  constraint vertical L8
  constraint horizontal L9
  constraint vertical L10
  constraint coincident L0 L8.end
  constraint coincident L7.start L10.end
  constraint horizontal L12
  constraint vertical L13
  constraint horizontal L14
  constraint vertical L15
  constraint coincident L9 L13.end
  constraint horizontal L16
  constraint vertical L17
  constraint horizontal L18
  constraint vertical L19
  constraint coincident L3 L17.end
  constraint horizontal L20
  constraint perpendicular L20 L21
  constraint parallel L20 L22
  constraint parallel L21 L23
  constraint coincident L24 P5
  constraint coincident L25 P5
  constraint coincident L0 L20.start
  constraint horizontal L26
  constraint perpendicular L26 L27
  constraint parallel L26 L28
  constraint parallel L27 L29
  constraint coincident L30 P4
  constraint coincident L31 P4
  constraint midpoint L5 L26.start
  constraint horizontal L32
  constraint perpendicular L32 L33
  constraint parallel L32 L34
  constraint parallel L33 L35
  constraint coincident L36 P4
  constraint coincident L37 P4
  constraint coincident L28 L32.start
  constraint coincident P4 P3
  constraint horizontal L38
  constraint perpendicular L38 L39
  constraint parallel L38 L40
  constraint parallel L39 L41
  constraint coincident L42 P5
  constraint coincident L43 P5
  constraint coincident L7 L38.start
  constraint coincident P5 P2
extrude "Extrude3" cut sketch "Sketch8" against normal blind 10 contours L0 L2 L3 L5 L17 L26 L28 L32 L33 L34 | L0 L2 L3 L4 L5 L16 L17 L18 L19 L26 L28 L32 L34 | L0 L2 L4 L19 L26 L28 L32 L34 L35 | L0 L2 L8 L15 L20 L22 L38 L39 L40 | L0 L2 L7 L8 L9 L12 L13 L14 L15 L20 L22 L38 L40 | L0 L2 L7 L9 L13 L20 L22 L38 L40 L41 bodies 2 in component "Component"
sketch "Sketch9" plane through (0, 0, 0) normal (0, -1, 0) x (1, 0, 0)
  line L0 (75.9, 62) -> (5.1, 62)
  line L1 (-30, 62) -> (-30, 15)
  line L2 (-30, 15) -> (1.5588, 15)
  line L3 (3.4412, 15) -> (77.5588, 15)
  line L4 (79.4412, 15) -> (111, 15)
  line L5 (111, 15) -> (111, 62)
  line L6 (5.1, 52) -> (2.9, 52)
  line L7 (-15.347, 37.6325) -> (-14.3209, 40.4516)
  line L8 (-14.3209, 40.4516) -> (-7.7431, 38.0574)
  line L9 (-7.7431, 38.0574) -> (-8.7691, 35.2384)
  line L10 (-8.7691, 35.2384) -> (-15.347, 37.6325)
  circle A0 centre (83, 28) radius 7.05
  line L11 (99.1615, 38.6711) -> (98.1354, 41.4902)
  line L12 (98.1354, 41.4902) -> (104.7133, 43.8843)
  line L13 (104.7133, 43.8843) -> (105.7393, 41.0652)
  line L14 (105.7393, 41.0652) -> (99.1615, 38.6711)
  line L15 (-24.7393, 41.0652) -> (-23.7133, 43.8843)
  line L16 (-23.7133, 43.8843) -> (-17.1354, 41.4902)
  line L17 (-17.1354, 41.4902) -> (-18.1615, 38.6711)
  line L18 (-18.1615, 38.6711) -> (-24.7393, 41.0652)
  circle A1 centre (-2, 28) radius 7.05
  line L19 (96.347, 37.6325) -> (89.7691, 35.2384)
  line L20 (89.7691, 35.2384) -> (88.7431, 38.0574)
  line L21 (88.7431, 38.0574) -> (95.3209, 40.4516)
  line L22 (95.3209, 40.4516) -> (96.347, 37.6325)
  circle A2 centre (56, 32.6) radius 7.05
  circle A3 centre (70, 46.6) radius 1.95
  circle A4 centre (22, 46.6) radius 1.95
  line L23 (1.5588, 15) -> (-0.2598, 18.15)
  line L24 (-0.2598, 18.15) -> (5.2598, 18.15)
  line L25 (5.2598, 18.15) -> (3.4412, 15)
  line L26 (77.5588, 15) -> (75.7402, 18.15)
  line L27 (75.7402, 18.15) -> (81.2598, 18.15)
  line L28 (81.2598, 18.15) -> (79.4412, 15)
  circle A5 centre (70, 56.6) radius 1.95
  circle A6 centre (22, 56.6) radius 1.95
  circle A7 centre (56, 51.6) radius 8.5
  line L29 (1.5, 52) -> (6.5, 52)
  line L30 (6.5, 52) -> (4, 56.3301)
  line L31 (4, 56.3301) -> (1.5, 52)
  line L32 (74.5, 52) -> (79.5, 52)
  line L33 (79.5, 52) -> (77, 56.3301)
  line L34 (77, 56.3301) -> (74.5, 52)
  line L35 (79.7598, 51.85) -> (77, 56.6301)
  line L36 (77, 56.6301) -> (74.2402, 51.85)
  line L37 (74.2402, 51.85) -> (79.7598, 51.85)
  line L38 (1.2402, 51.85) -> (6.7598, 51.85)
  line L39 (6.7598, 51.85) -> (4, 56.6301)
  line L40 (4, 56.6301) -> (1.2402, 51.85)
  line L41 (75.9, 52) -> (75.9, 62)
  line L42 (5.1, 62) -> (5.1, 52)
  line L43 (2.9, 52) -> (2.9, 62)
  line L44 (2.9, 62) -> (-30, 62)
  line L45 (111, 62) -> (78.1, 62)
  line L46 (78.1, 62) -> (78.1, 52)
  line L47 (78.1, 52) -> (75.9, 52)
  point P0 (2.5, 53.4434)
  point P1 (78.5, 53.4434)
  point P2 (4, 53.4434)
  point P3 (77, 53.4434)
  dimension "d155" = 0.15
  dimension "d156" = 0.15
extrude "Extrude4" cut sketch "Sketch9" against normal blind 5 contours L32 L33 L34 L35 L36 L37 L41 L46 L47 | L6 L29 L30 L31 L38 L39 L40 L42 L43 | L32 L34 L41 | L29 L30 L42 | L32 L33 L46 | L29 L31 L43 bodies 2 in component "Component"
delete_face "DeleteFace4" 1 faces at (1.9863, 5, 19.3003) on bodies 2 in component "Component"
delete_face "DeleteFace5" 1 faces at (4.4804, 5, 15.9) on bodies 2 in component "Component"
delete_face "DeleteFace6" 1 faces at (0.5196, 5, 15.9) on bodies 2 in component "Component"
component "Component" placed x (1, 0, 0) y (0, 0, 1) z (0, -1, 0) at (0, 34.0061, 0.0547)
component "Component" placed x (1, 0, 0) y (0, 0, 1) z (0, -1, 0) at (0, 114.0061, 0.0547)
equation "d5 = 42.00 mm + 20 mm"

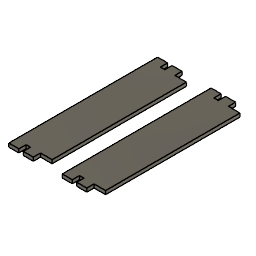
design "card-shuffler-platforms"
part number: 2026-07-28-16-04-37-564
part number: 2026-07-29-15-19-14-329
part number: 2026-07-29-15-19-15-565
Autodesk Fusion 360 part; units mm, degrees
sketch "Sketch1" plane through (0, 0, 0) normal (0, 0, 1) x (1, 0, 0)
  line L0 (0, 0) -> (25, 0)
  line L1 (25, 0) -> (25, 103)
  line L2 (25, 103) -> (0, 103)
  line L3 (0, 103) -> (0, 0)
  line L4 (0, 0) -> (2.25, 0)
  line L5 (0, 5) -> (25, 5)
  line L6 (0, 98) -> (25, 98)
  line L7 (0, 98) -> (7, 98)
  line L8 (7, 98) -> (7, 103)
  line L9 (7, 103) -> (0, 103)
  line L10 (0, 103) -> (0, 98)
  line L11 (7, 5) -> (0, 5)
  line L12 (0, 5) -> (0, 0)
  line L13 (0, 0) -> (7, 0)
  line L14 (7, 0) -> (7, 5)
  line L15 (10, 5) -> (17, 5)
  line L16 (17, 5) -> (17, 0)
  line L17 (17, 0) -> (10, 0)
  line L18 (10, 0) -> (10, 5)
  line L19 (10, 103) -> (17, 103)
  line L20 (17, 103) -> (17, 98)
  line L21 (17, 98) -> (10, 98)
  line L22 (10, 98) -> (10, 103)
  point P0 (25, 51.5)
  point P1 (25, 51.5)
  dimension "d1" = 25
  dimension "d2" = 103
  constraint horizontal L0
  constraint vertical L1
  constraint horizontal L2
  constraint vertical L3
  constraint coincident L0.start L3.end
  constraint coincident L0 L4.end
  constraint coincident L3 L5.start
  constraint coincident L1 L5.end
  constraint perpendicular L1 L5
  constraint coincident L3 L6.start
  constraint coincident L1 L6.end
  constraint perpendicular L1 L6
  constraint midpoint L1 P1
  constraint coincident P1 P0
  constraint horizontal L7
  constraint vertical L8
  constraint horizontal L9
  constraint vertical L10
  constraint horizontal L11
  constraint vertical L12
  constraint horizontal L13
  constraint vertical L14
  constraint coincident L5 L11.start
  constraint horizontal L15
  constraint vertical L16
  constraint horizontal L17
  constraint vertical L18
  constraint coincident L0 L16.end
  constraint coincident L5 L15.start
  constraint horizontal L19
  constraint vertical L20
  constraint horizontal L21
  constraint vertical L22
  constraint coincident L6 L20.end
  constraint coincident L2 L19.start
  measures "d1" distance of L0.start L0.end
  measures "d2" distance of L0.start L2.end
extrude "Extrude1" add sketch "Sketch1" along normal blind 2.5 contours L0 L3 L4 L5 L11 L12 L13 L14 | L1 L3 L5 L6 L7 L11 L15 L21 | L2 L3 L6 L7 L8 L9 L10 | L0 L5 L15 L16 L17 L18 | L2 L6 L19 L20 L21 L22 makes body 1
copy_body "CopyPasteBodies1" bodies 1 makes body 2
move_body "Move1" bodies 2 to x (1, 0, 0) y (0, 1, 0) z (0, 0, 1) at (37, 0, 0)
copy_body "Body->Comp1" bodies 1 removing the originals makes body 3 in component "Component"
copy_body "Body->Comp2" bodies 2 removing the originals makes body 4 in component "Component'"
component "Component" placed x (1, 0, 0) y (0, 1, 0) z (0, 0, 1) at (0, 0, 0)
component "Component'" placed x (1, 0, 0) y (0, 1, 0) z (0, 0, 1) at (0, 0, 0)

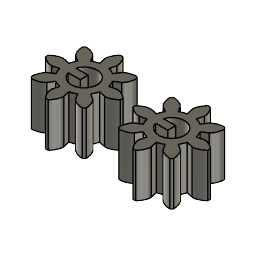
design "card-shuffler-driven-gears"
part number: 2026-07-29-20-17-55-869
part number: 2026-08-18-20-32-56-588
Autodesk Fusion 360 part; units mm, degrees